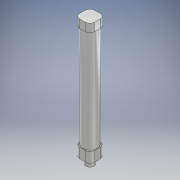
# Autodesk Inventor part: aircylinder16_100_part1_sa
Saved by Autodesk Inventor 2018 (Build 220112000, 112)
## iProperties
Created: 2018-03-06
Part Number: aircylinder16_100_part1_sa
Material: アルミニウム 6061-AHC
Document SubType Name: Modeling
Designer: shun
Density: 2.7 g/cm^3
Appearance: アルミニウム - ダーク
Author: shun
Autodesk Inventor part; units mm, degrees
ref_plane "YZ Plane" through (0, 0, 0) normal (1, 0, 0) x (0, 1, 0)
ref_plane "XZ Plane" through (0, 0, 0) normal (0, 1, 0) x (-1, 0, 0)
ref_plane "XY Plane" through (0, 0, 0) normal (0, 0, 1) x (1, 0, 0)
sketch "スケッチ1" plane through (0, 0, 0) normal (0, 0, 1) x (1, 0, 0)
  line L0 (9.15, -9.15) -> (-9.15, -9.15)
  line L1 (-9.15, -9.15) -> (-9.15, 9.15)
  line L2 (-9.15, 9.15) -> (9.15, 9.15)
  line L3 (9.15, 9.15) -> (9.15, -9.15)
  line L4 (9.15, -9.15) -> (-9.15, 9.15) construction
  line L5 (-9.15, -9.15) -> (9.15, 9.15) construction
  point P0 (0, 0)
  dimension "d0" = 18.3
  dimension "d1" = 18.3
  constraints: 12 end point, 2 midpoint, 2 parallel, 1 horizontal, 1 perpendicular
  measures "d0" distance of L1.end L2.end
  measures "d1" distance of L0.end L1.end
extrude "押し出し1" add sketch "スケッチ1" along normal blind 12.5
sketch "スケッチ2" plane through (0, 0, 12.5) normal (0, 0, 1) x (1, 0, 0)
  circle A0 centre (0, 0) radius 8.75
  dimension "d4" = 17.5
  constraints: 1 centre point, 1 coincident
  measures "d4" diameter of A0
extrude "押し出し2" add sketch "スケッチ2" along normal blind 125
sketch "スケッチ3" plane through (0, 0, 137.5) normal (0, 0, 1) x (1, 0, 0)
  line L0 (-9.15, -9.15) -> (9.15, -9.15)
  line L1 (9.15, -9.15) -> (9.15, 9.15)
  line L2 (9.15, 9.15) -> (-9.15, 9.15)
  line L3 (-9.15, 9.15) -> (-9.15, -9.15)
  line L4 (-9.15, -9.15) -> (9.15, 9.15) construction
  line L5 (9.15, -9.15) -> (-9.15, 9.15) construction
  point P0 (0, 0)
  dimension "d7" = 18.3
  dimension "d8" = 18.3
  constraints: 12 end point, 2 midpoint, 2 parallel, 1 horizontal, 1 perpendicular
  measures "d7" distance of L2.end L1.end
  measures "d8" distance of L1.end L0.end
extrude "押し出し3" add sketch "スケッチ3" along normal blind 10
fillet "フィレット1" radius 6 4 edges at (9.15, 9.15, 142.5) (9.15, -9.15, 142.5) (-9.15, 9.15, 142.5) (-9.15, -9.15, 142.5)
fillet "フィレット2" radius 6 4 edges at (9.15, 9.15, 6.25) (9.15, -9.15, 6.25) (-9.15, 9.15, 6.25) (-9.15, -9.15, 6.25)
sketch "スケッチ4" plane through (0, 0, 0) normal (0, 0, -1) x (-1, 0, 0)
  circle A0 centre (0, 0) radius 5
  dimension "d13" = 10
  constraints: 1 centre point, 1 coincident
  measures "d13" diameter of A0
extrude "押し出し4" add sketch "スケッチ4" along normal blind 8
sketch "スケッチ5" plane through (0, 0, -8) normal (0, 0, -1) x (-1, 0, 0)
  circle A0 centre (0, 0) radius 2.5
  dimension "d16" = 5
  constraints: 1 centre point, 1 coincident
  measures "d16" diameter of A0
extrude "押し出し5" cut sketch "スケッチ5" against normal blind 100
